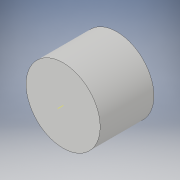
# Autodesk Inventor part: MountV01-CombinedWithCamera
Saved by Autodesk Inventor 2019.1 (Build 231200000, 200)
## iProperties
Created: 2018-11-03
Part Number: MountV01-CombinedWithCamera
Material: Generic
Document SubType Name: Modeling
Designer: steele
Density: 1 g/cm^3
Appearance: Default
Author: steele
Autodesk Inventor part; units mm, degrees
ref_plane "YZ Plane" through (0, 0, 0) normal (1, 0, 0) x (0, 1, 0)
ref_plane "XZ Plane" through (0, 0, 0) normal (0, 1, 0) x (-1, 0, 0)
ref_plane "XY Plane" through (0, 0, 0) normal (0, 0, 1) x (1, 0, 0)
sketch "Sketch1" plane through (0, 0, 0) normal (0, 0, 1) x (1, 0, 0)
  circle A0 centre (0, 0) radius 35
  dimension "d0" = 70
  constraints: 1 centre point, 1 coincident
  measures "d0" diameter of A0
extrude "Extrusion1" add sketch "Sketch1" along normal blind 50.8
sketch "Sketch2" plane through (0, 0, 0) normal (0, 0, -1) x (-1, 0, 0)
  circle A0 centre (0, 0) radius 31
  circle A1 centre (0, 0) radius 24
  dimension "d3" = 62
  dimension "d4" = 48
  constraints: 2 centre point, 2 coincident
  measures "d3" diameter of A0
  measures "d4" diameter of A1
extrude "Extrusion2" cut sketch "Sketch2" against normal blind 2
equation "\"d3\" = ringOuterDiam + ringDiamGap"
equation "\"d4\" = ringInnerDiam - ringDiamGap"
equation "\"ringOuterDiam\" = 60"
equation "\"ringInnerDiam\" = 50"
equation "\"ringThickness\" = 1.5"
equation "\"ringDiamGap\" = 2"
body "Solid1"
